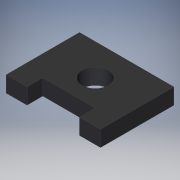
# Autodesk Inventor part: electromagnet_mnt_p1
Saved by Autodesk Inventor 2017 (Build 210142000, 142)
## iProperties
Created: 2018-03-20
Part Number: electromagnet_mnt_p1
Material: Generic
Document SubType Name: Modeling
Designer: Nic
Density: 1 g/cm^3
Appearance: Default
Author: Nic
Autodesk Inventor part; units mm, degrees
ref_plane "YZ Plane" through (0, 0, 0) normal (1, 0, 0) x (0, 1, 0)
ref_plane "XZ Plane" through (0, 0, 0) normal (0, 1, 0) x (-1, 0, 0)
ref_plane "XY Plane" through (0, 0, 0) normal (0, 0, 1) x (1, 0, 0)
sketch "Sketch1" plane through (0, 0, 0) normal (0, 0, 1) x (1, 0, 0)
  circle A0 centre (0, 0) radius 2.5
  line L0 (-9, 6) -> (9, 6)
  line L1 (9, 6) -> (9, -5)
  line L2 (-9, -6.6787) -> (-9, 6)
  line L3 (0, 0) -> (9, 0) construction
  line L4 (0, 0) -> (0, 6) construction
  line L5 (-9, -6.6787) -> (-9, -8)
  line L6 (-9, -8) -> (-5, -8)
  line L7 (-5, -8) -> (-5, -5)
  line L8 (9, -5) -> (9, -8)
  line L9 (5, -8) -> (5, -5)
  line L10 (5, -8) -> (9, -8)
  line L11 (5, -5) -> (-5, -5)
  dimension "d1" = 5
  dimension "d3" = 6
  dimension "d6" = 4
  dimension "d8" = 18
  dimension "d9" = 5
  dimension "d10" = 3
  constraints: 24 end point, 5 perpendicular, 3 symmetric about line, 2 horizontal, 2 parallel, 1 centre point, 1 coincident, 1 midpoint, 1 point on line, 1 vertical, 1 other
  measures "d1" diameter of A0
  measures "d3" distance from line of point (0, 0) L0
  measures "d6" distance of L5.end L6.end
  measures "d8" distance of L0.start L0.end
  measures "d9" distance from line of point (0, 0) L11
  measures "d10" distance of L9.start L9.end
extrude "Extrusion1" add sketch "Sketch1" along normal blind 3
body "Solid1"
